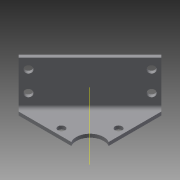
# Autodesk Inventor part: Bearing Mount 3 v1
Saved by Autodesk Inventor 2013 (Build 170138000, 138)
## iProperties
Created: 2013-01-18
Part Number: Bearing Mount 3 v1
Material: Generic
Document SubType Name: Sheet Metal
Designer: actoennies
Density: 1 g/cm^3
Sheet Metal Rule: Default
Author: actoennies
Autodesk Inventor part; units mm, degrees
ref_plane "YZ Plane" through (0, 0, 0) normal (1, 0, 0) x (0, 1, 0)
ref_plane "XZ Plane" through (0, 0, 0) normal (0, 1, 0) x (-1, 0, 0)
ref_plane "XY Plane" through (0, 0, 0) normal (0, 0, 1) x (1, 0, 0)
sketch "Sketch1" plane through (0, 0, 0) normal (0, 1, 0) x (-1, 0, 0)
  circle A0 centre (0, 0) radius 26.543 construction
  circle A1 centre (0, 26.543) radius 3.302
  circle A2 centre (26.543, 0) radius 3.302
  circle A3 centre (0, -26.543) radius 3.302
  circle A4 centre (-26.543, 0) radius 3.302
  circle A5 centre (0, 0) radius 12.7
  line L0 (0, 0) -> (-8.4134, 0) construction
  line L1 (10.9985, 6.35) -> (59.8338, 6.35)
  line L2 (-6.35, -10.9985) -> (-6.35, -59.8338)
  line L3 (59.8338, 6.35) -> (-6.35, -59.8338)
  dimension "d0" = 53.086
  dimension "d1" = 6.604
  dimension "d2" = 6.604
  dimension "d3" = 6.604
  dimension "d4" = 6.604
  dimension "d5" = 25.4
  dimension "d8" = 6.35
  dimension "d9" = 0
  dimension "d10" = 6.35
  dimension "d11" = 6.35
  dimension "d12" = 45
  dimension "d13" = 19.05
  measures "d0" diameter of A0
  measures "d1" diameter of A1
  measures "d2" diameter of A2
  measures "d3" diameter of A3
  measures "d4" diameter of A4
  measures "d5" diameter of A5
  measures "d8" distance from line of L2 A3.centre
  measures "d9" horizontal distance of A3.centre point (0, 0)
  measures "d10" distance from line of point (0, 0) L1
  measures "d11" distance from line of L1 A2.centre
  measures "d12" angle of L0 L3
  measures "d13" distance from line of A2.centre L3
extrude "Plate1" add sketch "Sketch1" along normal blind 3.175 contours A5 L1 L3 L2
sketch "Sketch2" plane through (-62.0788, 6.35, 4.1049) normal (-0.7071068, 0, -0.7071068) x (0, -1, 0)
  line L0 (0, -93.598) -> (0, 0)
  line L1 (0, 0) -> (-38.1, 0)
  line L2 (-38.1, 0) -> (-38.1, -93.598)
  line L3 (-38.1, -93.598) -> (0, -93.598)
  constraints: 6 end point, 1 horizontal, 1 perpendicular, 1 vertical
edge flange "Flange1" height 44.45 angle 90 thickness 3.175 bend radius 3.175 thickness toward (-0.7071068, 0, -0.7071068) relief straight relief width 3.175 relief depth 1.5875 edges at (-26.7419, 3.175, -26.7419) wall of the first edge with corners at (4.1049, 6.35, -62.0788) (-62.0788, 6.35, 4.1049) (-62.0788, 44.45, 4.1049) (4.1049, 44.45, -62.0788)
bend "Bend1"
corner "Corner1"
sketch "Sketch3" plane through (4.1049, 6.35, -62.0788) normal (0.7071068, 0, 0.7071068) x (0.7071068, 0, -0.7071068)
  line L0 (0, 38.1) -> (-93.598, 38.1) projected
  line L1 (0, 38.1) -> (0, 0) projected
  line L2 (-93.598, 38.1) -> (-93.598, 0) projected
  line L3 (-93.598, 0) -> (0, 0) projected
  circle A0 centre (-87.248, 28.575) radius 3.3782
  circle A1 centre (-6.35, 28.575) radius 3.3782
  circle A2 centre (-6.35, 9.525) radius 3.3782
  circle A3 centre (-87.248, 9.525) radius 3.3782
  point P0 (-46.799, -6.35)
  dimension "d35" = 93.598
  dimension "d36" = 6.7564
  dimension "d37" = 6.7564
  dimension "d38" = 6.7564
  dimension "d39" = 6.7564
  dimension "d40" = 6.35
  dimension "d41" = 9.525
  dimension "d42" = 9.525
  dimension "d43" = 6.35
  dimension "d44" = 9.525
  dimension "d45" = 9.525
  dimension "d47" = 6.35
  dimension "d48" = 6.35
  constraints: 4 centre point
  measures "d35" distance between parallel lines of L1 L2
  measures "d36" diameter of A0
  measures "d37" diameter of A1
  measures "d38" diameter of A2
  measures "d39" diameter of A3
  measures "d40" distance from line of L1 A1.centre
  measures "d41" distance from line of L0 A1.centre
  measures "d42" distance from line of L3 A2.centre
  measures "d43" distance from line of L1 A2.centre
  measures "d44" distance from line of L0 A0.centre
  measures "d45" distance from line of L3 A3.centre
  measures "d47" distance from line of L2 A0.centre
  measures "d48" distance from line of L2 A3.centre
extrude "Cut3" cut sketch "Sketch3" against normal blind 3.175 contours A0 | A1 | A2 | A3
equation "\"d49\" = Thickness"
equation "\"d15\" = BendReliefWidth"
equation "\"d16\" = BendReliefDepth"
equation "\"d17\" = MinimumRemnant"
equation "\"d18\" = BendRadius"
equation "\"d21\" = BendRadius"
equation "\"d22\" = CornerReliefSize"
equation "\"d23\" = GapSize"
equation "\"d24\" = JacobiRadiusSize"
equation "\"BendRadius\" = Thickness"
equation "\"BendReliefWidth\" = Thickness"
equation "\"BendReliefDepth\" = 0.5 * Thickness"
equation "\"CornerReliefSize\" = 4 * Thickness"
equation "\"MinimumRemnant\" = 2 * Thickness"
equation "\"TransitionRadius\" = BendRadius"
equation "\"JacobiRadiusSize\" = BendRadius"
equation "\"GapSize\" = Thickness"
equation "\"d14\" = BendRadius"
equation "\"Thickness\" = 3.175"
body "Solid1"
